e3dSecureFan (Autodesk Fusion 360 design; units mm, degrees)
Autodesk Fusion 360 part; units mm, degrees
mesh "Mesh1" [no effect]
sketch "Sketch1" plane through (0, 0, 0) normal (0, 1, 0) x (1, 0, 0)
  circle A0 centre (0, 0) radius 11
  line L0 (17.5, 20) -> (-17.5, 20)
  line L1 (-17.5, 20) -> (-17.5, -20)
  line L2 (-17.5, -20) -> (17.5, -20)
  line L3 (17.5, -20) -> (17.5, 20)
  line L4 (17.5, 20) -> (-17.5, -20) construction
  line L5 (-17.5, 20) -> (17.5, -20) construction
  line L6 (-17.5, 14.6272) -> (-17.5, -7.5023)
  line L7 (17.5, -13.8287) -> (17.5, 14.6272)
  line L8 (-17.5, -7.5023) -> (-8.0446, -7.5023)
  line L9 (-8.0446, -7.5023) -> (-8.0446, 7.5023)
  line L10 (-8.0446, 7.5023) -> (-17.5, 7.5023)
  line L11 (-17.5, 7.5023) -> (-17.5, -7.5023)
  line L12 (14.0701, 20) -> (14.0701, -20)
  dimension "d1" = 22
  dimension "d2" = 40
  dimension "d3" = 35
  constraint coincident A0.centre origin
  constraint perpendicular L0 L1
  constraint parallel L0 L2
  constraint parallel L1 L3
  constraint horizontal L0
  constraint coincident L4 A0.centre
  constraint coincident L5 A0.centre
  constraint vertical L6
  constraint vertical L7
  constraint coincident L3 A0.centre
  constraint coincident L1
  constraint horizontal L8
  constraint vertical L9
  constraint horizontal L10
  constraint vertical L11
  constraint coincident L0
  constraint coincident L2 A0.centre
  constraint perpendicular L2 L12
  measures "d1" diameter of A0
  measures "d2" distance of A0.centre
extrude "Extrude1" add sketch "Sketch1" along normal blind 40 contours A0 L0 L1 L2 L6 L8 L10 L12 | A0 L1 L6 L8 L10 L11 | L0 L2 L3 L7 L12
sketch "Sketch2" plane through (17.5, 0, 0) normal (1, 0, 0) x (0, 0, -1)
  line L0 (-20, 0) -> (20, 0)
  line L1 (20, 0) -> (20, 40)
  line L2 (20, 40) -> (-20, 40)
  line L3 (-20, 40) -> (-20, 0)
  line L4 (-20, 40) -> (20, 0) construction
  line L5 (20, 40) -> (-20, 0) construction
  circle A0 centre (0, 20) radius 18.7883
  circle A1 centre (0, 20) radius 12.5
  line L6 (16, 36) -> (-16, 36) construction
  line L7 (-16, 36) -> (-16, 4) construction
  line L8 (-16, 4) -> (16, 4) construction
  line L9 (16, 4) -> (16, 36) construction
  line L10 (16, 36) -> (-16, 4) construction
  line L11 (-16, 36) -> (16, 4) construction
  circle A2 centre (-16, 36) radius 2
  circle A3 centre (16, 36) radius 2
  circle A4 centre (-16, 4) radius 2
  circle A5 centre (16, 4) radius 2
  circle A6 centre (-16, 36) radius 3.1623
  circle A7 centre (16, 36) radius 3.5
  circle A8 centre (-16, 4) radius 3.5
  circle A9 centre (16, 4) radius 3.5
  dimension "d21" = 25
  dimension "d28" = 32
  dimension "d29" = 32
  dimension "d30" = 4
  dimension "d31" = 4
  dimension "d32" = 4
  dimension "d33" = 4
  dimension "d37" = 6.3246
  dimension "d38" = 7
  dimension "d39" = 7
  dimension "d40" = 7
  constraint midpoint L4 origin
  constraint concentric A0 A1
  constraint perpendicular L6 L7
  constraint parallel L6 L8
  constraint parallel L7 L9
  constraint horizontal L6
  constraint coincident L10 origin
  constraint coincident L11 origin
  constraint concentric A2 A6
  constraint concentric A3 A7
  constraint concentric A4 A8
  constraint concentric A5 A9
  measures "d21" diameter of A1
  measures "d29" distance of origin
  measures "d30" diameter of A2
  measures "d31" diameter of A3
  measures "d32" diameter of A4
  measures "d33" diameter of A5
  measures "d37" diameter of A6
  measures "d38" diameter of A7
  measures "d39" diameter of A8
  measures "d40" diameter of A9
extrude "Extrude2" cut sketch "Sketch2" against normal blind 2 contours A0 | A1
sketch "Sketch3" plane through (0, 0, -20) normal (0, 0, -1) x (-1, 0, 0)
  line L0 (-17.5, 0) -> (17.5, 0)
  line L1 (17.5, 0) -> (17.5, 40)
  line L2 (17.5, 40) -> (-17.5, 40)
  line L3 (-17.5, 40) -> (-17.5, 0)
  circle A0 centre (12, 25) radius 1.65
  circle A1 centre (12, 15) radius 1.65
  dimension "d8" = 3.3
  dimension "d9" = 3.3
  measures "d8" diameter of A0
  measures "d9" diameter of A1
extrude "Extrude3" cut sketch "Sketch3" against normal blind 53 contours A0 | A1
extrude "Extrude4" cut sketch "Sketch1" along normal blind 68 contours A0 L9 | A0 L1 L6 L8 L10 L11 picked at (-9.3364, 0.638)
extrude "Extrude5" cut sketch "Sketch1" along normal blind 7 contours A0 L0 L1 L2 L6 L8 L10 L12
extrude "Extrude6" cut sketch "Sketch1" along normal blind 40 and the other way blind -33 contours A0 L0 L1 L2 L6 L8 L10 L12
extrude "Extrude7" add sketch "Sketch2" along normal blind 6 contours L0 L1 L2 L3 | A2 | A3 | A4 | A5 | A6 | A7 | A8 | A9
extrude "Extrude8" cut sketch "Sketch2" against normal blind 42 contours A1
fillet "Fillet1" radius 2.5 1 edges at (15.5, 24.5202, 11.6541)
fillet "Fillet2" radius 9.5 1 edges at (15.5, 26.7941, 17.5168)
fillet "Fillet3" radius 11 1 edges at (14.0701, 33, 0)
fillet "Fillet4" radius 11 1 edges at (14.0701, 7, 0)
extrude "Extrude9" cut sketch "Sketch2" along normal blind 11 and the other way blind 14 contours A2 | A3 | A4 | A5
extrude "Extrude10" cut sketch "Sketch2" against normal blind 22 contours A6 | A7 | A8 | A9
